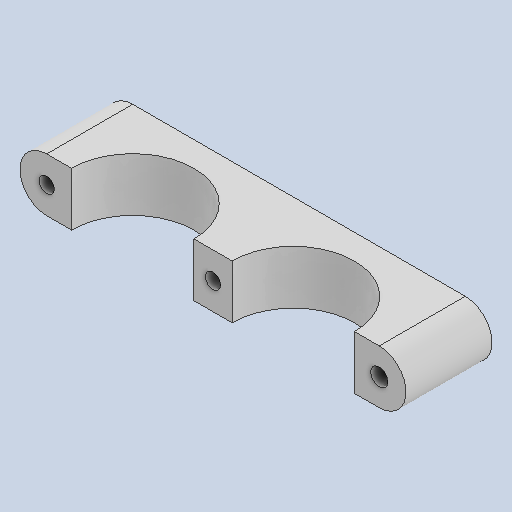
# Autodesk Inventor part: Uchwyt_silnika_podwojny
Saved by Autodesk Inventor 2022 (Build 260153000, 153)
## iProperties
Created: 2023-02-06
Part Number: Uchwyt_silnika_podwojny
Material: Generic
Document SubType Name: Modeling
Designer: Kamil
Density: 1 g/cm^3
Appearance: Default
Author: Kamil
Autodesk Inventor part; units mm, degrees
ref_plane "YZ Plane" through (0, 0, 0) normal (1, 0, 0) x (0, 1, 0)
ref_plane "XZ Plane" through (0, 0, 0) normal (0, 1, 0) x (-1, 0, 0)
sketch "Sketch1" plane through (0, 0, 0) normal (0, 0, 1) x (1, 0, 0)
  circle A0 centre (-88.75, 237.1618) radius 2 projected
  circle A1 centre (-45.25, 302.7734) radius 2 projected
  circle A2 centre (-88.75, 302.7734) radius 2 projected
  circle A3 centre (-45.25, 237.1618) radius 2 projected
  circle A4 centre (-46.75, 361.06) radius 2 projected
  circle A5 centre (-40.75, 400) radius 23.3333 projected
  line L0 (-53.25, 186.7791) -> (-53.25, -39) projected
  arc A6 (-53.25, -39) -> (-46.25, -46) centre (-46.25, -39) ccw projected
  line L1 (1.25, -46) -> (-46.25, -46) projected
  arc A7 (1.25, -46) -> (8.9167, 45.3566) centre (1.25, 0) ccw projected
  arc A8 (7.25, 47.3286) -> (8.9167, 45.3566) centre (9.25, 47.3286) ccw projected
  line L2 (7.25, 400) -> (7.25, 47.3286) projected
  arc A9 (7.25, 400) -> (-27.0387, 446) centre (-40.75, 400) ccw projected
  line L3 (-85.75, 446) -> (-27.0387, 446) projected
  circle A10 centre (-85.75, 438.7) radius 2 projected
  circle A11 centre (-85.75, 361.06) radius 2 projected
  circle A12 centre (-46.75, 438.7) radius 2 projected
  circle A13 centre (10.9583, -29.879) radius 2.1 projected
  circle A14 centre (32.6667, 0) radius 2.1 projected
  circle A15 centre (-24.1666, -18.4663) radius 2.1 projected
  circle A16 centre (10.9583, 29.879) radius 2.1 projected
  circle A17 centre (-24.1666, 18.4663) radius 2.1 projected
  circle A18 centre (1.25, 0) radius 23.3333 projected
  circle A19 centre (-1.75, 302.7734) radius 2.25 projected
  circle A20 centre (-1.75, 237.1618) radius 2.25 projected
  circle A21 centre (-43.75, 127.6736) radius 2 projected
  circle A22 centre (-4.75, -38.7) radius 2 projected
  circle A23 centre (-4.75, 38.94) radius 2 projected
  circle A24 centre (-4.75, 127.6736) radius 2 projected
  circle A25 centre (-43.75, -38.7) radius 2 projected
  circle A26 centre (-43.75, 38.94) radius 2 projected
  line L4 (-88.75, 237.1618) -> (-95.75, 237.1618)
  line L5 (-1.75, 237.1618) -> (5.25, 237.1618)
  circle A27 centre (-88.75, 237.1618) radius 7
  circle A28 centre (-1.75, 237.1618) radius 7
  line L6 (-88.75, 230.1618) -> (-1.75, 230.1618)
  line L7 (-88.75, 244.1618) -> (-1.75, 244.1618)
  circle A29 centre (-9.3333, 400) radius 2.1 projected
  circle A30 centre (-31.0417, 429.879) radius 2.1 projected
  circle A31 centre (-31.0417, 370.121) radius 2.1 projected
  circle A32 centre (-66.1666, 418.4663) radius 2.1 projected
  circle A33 centre (-66.1666, 381.5337) radius 2.1 projected
  arc A34 (-95.75, 226.7791) -> (-85.75, 216.7791) centre (-85.75, 226.7791) ccw projected
  line L8 (-85.75, 216.7791) -> (-83.25, 216.7791) projected
  arc A35 (-53.25, 186.7791) -> (-83.25, 216.7791) centre (-83.25, 186.7791) ccw projected
  arc A36 (-85.75, 446) -> (-95.75, 436) centre (-85.75, 436) ccw projected
  line L9 (-95.75, 226.7791) -> (-95.75, 436) projected
  point P0 (0, 0)
  dimension "d0" = 7
  dimension "d1" = 7
  constraints: 8 end point, 6 point on circle, 2 centre point, 2 coincident, 2 horizontal, 1 parallel, 1 tangent
  measures "d0" distance of L4.start L4.end
  measures "d1" distance of L5.start L5.end
ref_plane "Work Plane1" through (-48.25, 120.3736, 22.5) normal (0, 0, -1) x (0, 1, 0)
extrude "Extrusion1" add sketch "Sketch1" along normal up to surface (22.5 mm away) contours A27 | L7 A28 L6 A27 | A28
sketch "Sketch2" plane through (-88.75, 230.1618, 0) normal (0, -1, 0) x (1, 0, 0)
  circle A0 centre (22.5, 22.5) radius 16 projected
  circle A1 centre (64.5, 22.5) radius 16 projected
  line L0 (0, 22.5) -> (87, 22.5) projected
  line L1 (0, 0) -> (0, 22.5) projected
  line L2 (0, 0) -> (87, 0) projected
  line L3 (87, 0) -> (87, 22.5) projected
  point P0 (88.75, 0)
  point P1 (80.5, 22.5)
  point P2 (48.5, 22.5)
  point P3 (38.5, 22.5)
  point P4 (6.5, 22.5)
extrude "Extrusion2" cut sketch "Sketch2" against normal through all contours A0 L0 | L0 A1 picked at (22.9879, 15.9292) picked at (60.5079, 16.4106)
body "Solid1"
